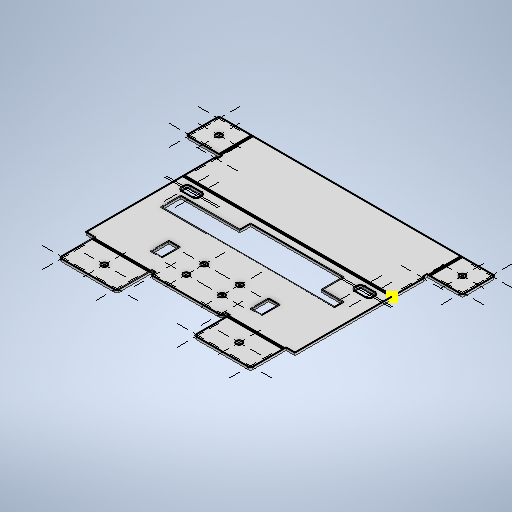
# Autodesk Inventor part: body_top_frame
Saved by Autodesk Inventor 2026.1 (Build 301233000, 233)
## iProperties
Created: 2025-08-15
Part Number: body_top_frame
Material: Generic
Document SubType Name: Modeling
Designer: chris
Density: 1 g/cm^3
Appearance: Default
Author: chris
Autodesk Inventor part; units mm, degrees
ref_plane "YZ Plane" through (0, 0, 0) normal (1, 0, 0) x (0, 1, 0)
ref_plane "XZ Plane" through (0, 0, 0) normal (0, 1, 0) x (-1, 0, 0)
ref_plane "XY Plane" through (0, 0, 0) normal (0, 0, 1) x (1, 0, 0)
sketch "Sketch1" plane through (0, 0, 0) normal (0, 1, 0) x (-1, 0, 0)
  line L0 (112, 55.3296) -> (80, 55.3296)
  line L1 (117.1396, -39.0893) -> (117.1396, -20.8993)
  line L2 (117, -0.4496) -> (0, -0.4496)
  line L3 (36.5, 55.3296) -> (5, 55.3296)
  line L4 (-0.1396, -20.8993) -> (-0.1396, -39.0893)
  circle A0 centre (48.25, 46.69) radius 1.55
  circle A1 centre (48.25, 36.69) radius 1.55
  circle A2 centre (68.25, 46.69) radius 1.55
  circle A3 centre (68.25, 36.69) radius 1.55
  line L5 (83.46, 35.26) -> (83.46, 45.26)
  line L6 (89.46, 35.26) -> (83.46, 35.26)
  line L7 (89.46, 45.26) -> (89.46, 35.26)
  line L8 (83.46, 45.26) -> (89.46, 45.26)
  line L9 (33.54, 45.26) -> (33.54, 35.26)
  line L10 (27.54, 45.26) -> (33.54, 45.26)
  line L11 (27.54, 35.26) -> (27.54, 45.26)
  line L12 (33.54, 35.26) -> (27.54, 35.26)
  line L13 (108, 21) -> (108, 10)
  line L14 (11, 21) -> (108, 21)
  line L15 (11, 16) -> (11, 21)
  line L16 (23, 16) -> (11, 16)
  line L17 (23, 4) -> (23, 16)
  line L18 (75, 4) -> (23, 4)
  line L19 (75, 10) -> (75, 4)
  line L20 (108, 10) -> (75, 10)
  arc A4 (112, 5.5) -> (110, 7.5) centre (110, 5.5) ccw
  line L21 (104, 7.5) -> (110, 7.5)
  arc A5 (110, 2.5) -> (112, 4.5) centre (110, 4.5) ccw
  line L22 (110, 2.5) -> (104, 2.5)
  arc A6 (102, 4.5) -> (104, 2.5) centre (104, 4.5) ccw
  line L23 (102, 4.5) -> (102, 5.5)
  arc A7 (104, 7.5) -> (102, 5.5) centre (104, 5.5) ccw
  arc A8 (15, 5.5) -> (13, 7.5) centre (13, 5.5) ccw
  line L24 (7, 7.5) -> (13, 7.5)
  arc A9 (13, 2.5) -> (15, 4.5) centre (13, 4.5) ccw
  line L25 (13, 2.5) -> (7, 2.5)
  arc A10 (5, 4.5) -> (7, 2.5) centre (7, 4.5) ccw
  line L26 (5, 4.5) -> (5, 5.5)
  arc A11 (7, 7.5) -> (5, 5.5) centre (7, 5.5) ccw
  line L27 (112, 5.5) -> (112, 4.5)
  line L28 (15, 5.5) -> (15, 4.5)
  circle A12 centre (20.5, 64.8743) radius 1.55
  circle A13 centre (96, 64.8743) radius 1.55
  circle A14 centre (-9.6843, -29.9943) radius 1.55
  circle A15 centre (126.6843, -29.9943) radius 1.55
  arc A16 (0, -17.8993) -> (1, -18.8993) centre (1, -17.8993) ccw
  arc A17 (116, -18.8993) -> (117, -17.8993) centre (116, -17.8993) ccw
  line L29 (115.94, -18.8993) -> (116, -18.8993)
  arc A18 (135.7793, -21.8993) -> (134.7793, -20.8993) centre (134.7793, -21.8993) ccw
  arc A19 (134.7793, -39.0893) -> (135.7793, -38.0893) centre (134.7793, -38.0893) ccw
  line L30 (134.7793, -39.0893) -> (-17.7793, -39.0893)
  arc A20 (-18.7793, -38.0893) -> (-17.7793, -39.0893) centre (-17.7793, -38.0893) ccw
  arc A21 (-17.7793, -20.8993) -> (-18.7793, -21.8993) centre (-17.7793, -21.8993) ccw
  line L31 (-17.7793, -20.8993) -> (1.06, -20.8993)
  arc A22 (39.5, 56.69) -> (38.5, 55.69) centre (39.5, 55.69) ccw
  line L32 (39.5, 56.69) -> (77, 56.69)
  arc A23 (78, 55.69) -> (77, 56.69) centre (77, 55.69) ccw
  arc A24 (81, 73.9693) -> (80, 72.9693) centre (81, 72.9693) ccw
  arc A25 (112, 72.9693) -> (111, 73.9693) centre (111, 72.9693) ccw
  arc A26 (6, 73.9693) -> (5, 72.9693) centre (6, 72.9693) ccw
  arc A27 (36.5, 72.9693) -> (35.5, 73.9693) centre (35.5, 72.9693) ccw
  line L33 (36.5, 72.9693) -> (36.5, 54.13)
  line L34 (6, 73.9693) -> (35.5, 73.9693)
  line L35 (38.5, 55.69) -> (38.5, 54.13)
  line L36 (38.5, 54.13) -> (36.5, 54.13)
  line L37 (5, 54.13) -> (5, 72.9693)
  line L38 (5, 54.13) -> (0, 54.13)
  line L39 (0, -17.8993) -> (0, 54.13)
  line L40 (81, 73.9693) -> (111, 73.9693)
  line L41 (112, 54.13) -> (112, 72.9693)
  line L42 (117, 54.13) -> (112, 54.13)
  line L43 (78, 54.13) -> (78, 55.69)
  line L44 (80, 72.9693) -> (80, 54.13)
  line L45 (80, 54.13) -> (78, 54.13)
  line L46 (117, 54.13) -> (117, -17.8993)
  line L47 (-18.7793, -38.0893) -> (-18.7793, -21.8993)
  line L48 (135.7793, -21.8993) -> (135.7793, -38.0893)
  line L49 (115.94, -20.8993) -> (134.7793, -20.8993)
  line L50 (115.94, -20.8993) -> (115.94, -18.8993)
  line L51 (1, -18.8993) -> (1.06, -18.8993)
  line L52 (1.06, -18.8993) -> (1.06, -20.8993)
  line L53 (-0.5893, -39.0893) -> (-0.5893, -20.8993)
  line L54 (117.5893, -20.8993) -> (117.5893, -39.0893)
  line L55 (0.31, -20.8993) -> (0.31, -39.0893)
  line L56 (116.69, -39.0893) -> (116.69, -20.8993)
  line L57 (5, 55.7793) -> (36.5, 55.7793)
  line L58 (117, -0.8993) -> (0, -0.8993)
  line L59 (80, 55.7793) -> (112, 55.7793)
  line L60 (36.5, 54.88) -> (5, 54.88)
  line L61 (0, 0) -> (117, 0)
  line L62 (112, 54.88) -> (80, 54.88)
  constraints: 126 end point, 54 tangent, 40 point on circle, 33 horizontal, 30 point on line, 30 vertical, 28 centre point, 28 perpendicular, 27 parallel, 25 equal radius, 2 collinear, 155 other
extrude "Extrusion1" add sketch "Sketch1" against normal blind 1.5
body "Solid1"
